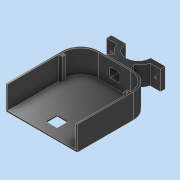
# Autodesk Inventor part: Part2
Saved by Autodesk Inventor 2022 (Build 260153000, 153)
## iProperties
Created: 2022-09-15
Part Number: Part2
Material: Generic
Document SubType Name: Modeling
Designer: aleal
Density: 1 g/cm^3
Appearance: Glossy - Black
Author: aleal
Autodesk Inventor part; units mm, degrees
ref_plane "YZ Plane" through (0, 0, 0) normal (1, 0, 0) x (0, 1, 0)
ref_plane "XZ Plane" through (0, 0, 0) normal (0, 1, 0) x (-1, 0, 0)
sketch "Sketch1" plane through (0, 0, 0) normal (0, 1, 0) x (-1, 0, 0)
  line L0 (0, 0) -> (146, 0)
  line L1 (146, 0) -> (146, -113)
  line L2 (146, -113) -> (0, -113)
  line L3 (0, -113) -> (0, 0)
  dimension "d0" = 146
  dimension "d1" = 113
  constraints: 8 end point, 2 parallel, 1 horizontal, 1 perpendicular
  measures "d0" distance of L1.end L2.end
  measures "d1" distance of L0.end L1.end
extrude "Extrusion1" add sketch "Sketch1" along normal blind 50
sketch "Sketch2" plane through (0, 50, 0) normal (0, 1, 0) x (1, 0, 0)
  line L0 (-146, 0) -> (0, 0) projected
  line L1 (-143, 0) -> (-3, 0)
  line L2 (-3, 0) -> (-3, 72.5)
  line L3 (-40.5, 110) -> (-105.5, 110)
  line L4 (-143, 72.5) -> (-143, 0)
  line L5 (-146, 113) -> (-146, 0) projected
  arc A0 (-105.5, 110) -> (-143, 72.5) centre (-105.5, 72.5) ccw
  arc A1 (-3, 72.5) -> (-40.5, 110) centre (-40.5, 72.5) ccw
  point P0 (-3, 110)
  point P1 (-143, 110)
  dimension "d4" = 140
  dimension "d5" = 110
  dimension "d6" = 3
  dimension "d19" = 37.5
  constraints: 8 end point, 5 point on line, 4 point on circle, 4 tangent, 2 centre point, 2 parallel, 1 equal radius, 1 horizontal, 1 perpendicular
  measures "d4" distance of point (-143, 110) point (-3, 110)
  measures "d5" distance of point (-3, 110) L1.end
  measures "d6" distance between parallel lines of L5 L4
  measures "d19" radius of A0
extrude "Extrusion2" cut sketch "Sketch2" against normal blind 47
ref_plane "Work Plane1" through (0, 45, 0) normal (0, 1, 0) x (1, 0, 0)
sketch "Sketch3" plane through (0, 45, 0) normal (0, 1, 0) x (1, 0, 0)
  arc A0 (-98.4, 158.6) -> (-47.6, 158.6) centre (-73, 158.6) ccw
  line L0 (0, 113) -> (-146, 113) projected
  arc A1 (-108.4, 158.6) -> (-37.6, 158.6) centre (-73, 158.6) ccw
  line L1 (-108.4, 158.6) -> (-98.4, 158.6)
  line L2 (-47.6, 158.6) -> (-37.6, 158.6)
  line L3 (-108.4, 158.6) -> (-128.4, 158.6)
  line L4 (-128.4, 158.6) -> (-128.4, 148.6)
  line L5 (-128.4, 148.6) -> (-106.9582, 148.6)
  line L6 (-37.6, 158.6) -> (-17.6, 158.6)
  line L7 (-17.6, 158.6) -> (-17.6, 148.6)
  line L8 (-17.6, 148.6) -> (-39.0418, 148.6)
  point P0 (0, 0)
  dimension "d10" = 50.8
  dimension "d11" = 45.6
  dimension "d12" = 10
  dimension "d13" = 20
  dimension "d14" = 10
  dimension "d15" = 20
  dimension "d16" = 10
  constraints: 16 end point, 6 point on circle, 4 horizontal, 4 perpendicular, 2 centre point
  measures "d10" diameter of A0
  measures "d11" distance from line of L0 A0.centre
  measures "d12" radial gap between concentric circles of A0 A1
  measures "d13" distance of L1.start L3.end
  measures "d14" distance of L3.end L4.end
  measures "d15" distance of L2.end L6.end
  measures "d16" distance of L6.end L7.end
extrude "Extrusion3" add sketch "Sketch3" against normal blind 40
fillet "Fillet1" radius 37.5 2 edges at (-146, 25, -113) (0, 25, -113)
sketch "Sketch5" plane through (0, 45, 0) normal (0, 1, 0) x (1, 0, 0)
  arc A0 (-106.9582, 148.6) -> (-39.0418, 148.6) centre (-73, 158.6) ccw projected
  line L0 (-37.5, 113) -> (-108.5, 113) projected
  line L1 (-93, 129.3911) -> (-93, 113)
  line L2 (-53, 129.3911) -> (-53, 113)
  point P0 (0, 0)
  constraints: 4 end point, 2 point on circle
extrude "Extrusion4" add sketch "Sketch5" against normal blind 40
fillet "Fillet2" radius 20 2 edges at (-93, 25, -113) (-53, 25, -113)
sketch "Sketch6" plane through (-146, 0, 0) normal (0, 0, 1) x (1, 0, 0)
  line L0 (0, 50) -> (37.5, 50) projected
  line L1 (0, 0) -> (0, 50) projected
  line L2 (0, 50) -> (0, 0)
  line L3 (0, 0) -> (146, 0) projected
  line L4 (0, 0) -> (146, 0)
  line L5 (146, 0) -> (146, 50) projected
  line L6 (146, 0) -> (146, 50)
  line L7 (143, 50) -> (146, 50) projected
  line L8 (146, 50) -> (143, 50)
  line L9 (143, 3) -> (3, 3) projected
  line L10 (143, 50) -> (143, 3)
  line L11 (143, 3) -> (3, 3)
  line L12 (3, 3) -> (3, 50)
  constraints: 14 end point, 4 perpendicular, 3 collinear, 1 point on line
extrude "Extrusion5" add sketch "Sketch6" along normal blind 40
sketch "Sketch7" plane through (-105.5, 50, -110) normal (0, 0, 1) x (1, 0, 0)
  line L0 (42.5, -33.5) -> (22.5, -33.5)
  line L1 (22.5, -33.5) -> (22.5, -13.5)
  line L2 (22.5, -13.5) -> (42.5, -13.5)
  line L3 (42.5, -13.5) -> (42.5, -33.5)
  line L4 (65, 0) -> (65, -47) projected
  line L5 (0, 0) -> (0, -47) projected
  line L6 (0, 0) -> (65, 0) projected
  line L7 (0, -47) -> (65, -47) projected
  point P0 (105.5, -50)
  dimension "d28" = 20
  dimension "d29" = 20
  dimension "d30" = 65
  dimension "d31" = 22.5
  dimension "d32" = 47
  dimension "d33" = 13.5
  constraints: 8 end point, 2 parallel, 1 horizontal, 1 perpendicular
  measures "d28" distance of L1.end L2.end
  measures "d29" distance of L0.end L1.end
  measures "d30" distance between parallel lines of L4 L5
  measures "d31" distance between parallel lines of L4 L3
  measures "d32" distance between parallel lines of L6 L7
  measures "d33" distance between parallel lines of L7 L0
extrude "Extrusion6" cut sketch "Sketch7" against normal blind 30 contours L0 L1 L2 L3
fillet "Fillet3" radius 2 4 edges at (-83, 36.5, -122.6257) (-83, 16.5, -122.6257) (-63, 36.5, -122.6257) (-63, 16.5, -122.6257)
sketch "Sketch8" plane through (0, 50, 0) normal (0, 1, 0) x (1, 0, 0)
  arc A0 (-105.5, 110) -> (-143, 72.5) centre (-105.5, 72.5) ccw projected
  line L0 (-143, 72.5) -> (-136, 72.5)
  line L1 (-136, 72.5) -> (-136, 65.5)
  line L2 (-136, 65.5) -> (-143, 65.5)
  line L3 (-143, 65.5) -> (-143, 72.5)
  arc A1 (-3, 72.5) -> (-40.5, 110) centre (-40.5, 72.5) ccw projected
  line L4 (-3, 72.5) -> (-10, 72.5)
  line L5 (-10, 72.5) -> (-10, 65.5)
  line L6 (-10, 65.5) -> (-3, 65.5)
  line L7 (-3, 65.5) -> (-3, 72.5)
  point P0 (0, 0)
  dimension "d37" = 7
  dimension "d38" = 7
  dimension "d39" = 7
  dimension "d40" = 7
  constraints: 16 end point, 4 parallel, 2 horizontal, 2 perpendicular
  measures "d37" distance of L1.end L2.end
  measures "d38" distance of L0.end L1.end
  measures "d39" distance of L6.end L5.end
  measures "d40" distance of L5.end L4.end
extrude "Extrusion7" add sketch "Sketch8" against normal blind 50
sketch "Sketch9" plane through (0, 50, 0) normal (0, 1, 0) x (1, 0, 0)
  circle A0 centre (-139.5, 69) radius 1.45
  line L0 (-136, 65.5) -> (-136, 72.5) projected
  line L1 (-136, 72.5) -> (-143, 72.5) projected
  circle A1 centre (-6.5, 69) radius 1.45
  line L2 (-10, 72.5) -> (-10, 65.5) projected
  line L3 (-3, 72.5) -> (-10, 72.5) projected
  point P0 (0, 0)
  dimension "d43" = 2.9
  dimension "d44" = 3.5
  dimension "d45" = 3.5
  dimension "d46" = 2.9
  dimension "d47" = 3.5
  dimension "d48" = 3.5
  constraints: 2 centre point
  measures "d43" diameter of A0
  measures "d44" distance from line of L0 A0.centre
  measures "d45" distance from line of L1 A0.centre
  measures "d46" diameter of A1
  measures "d47" distance from line of L2 A1.centre
  measures "d48" distance from line of L3 A1.centre
extrude "Extrusion8" cut sketch "Sketch9" against normal blind 50
sketch "Sketch10" plane through (-98.4, 45, -158.6) normal (0, 0, -1) x (-1, 0, 0)
  circle A0 centre (20, -20) radius 2.75
  circle A1 centre (-70.8, -20) radius 2.75
  line L0 (-50.8, -40) -> (-80.8, -40) projected
  line L1 (30, -40) -> (0, -40) projected
  line L2 (30, 0) -> (30, -40) projected
  line L3 (-80.8, 0) -> (-80.8, -40) projected
  point P0 (-98.4, -45)
  dimension "d54" = 5.5
  dimension "d55" = 5.5
  dimension "d56" = 20
  dimension "d57" = 20
  dimension "d58" = 10
  dimension "d59" = 10
  constraints: 2 centre point
  measures "d54" diameter of A0
  measures "d55" diameter of A1
  measures "d56" distance from line of L0 A1.centre
  measures "d57" distance from line of L1 A0.centre
  measures "d58" distance from line of L2 A0.centre
  measures "d59" distance from line of L3 A1.centre
extrude "Extrusion9" cut sketch "Sketch10" against normal blind 10
sketch "Sketch11" plane through (0, 3, 0) normal (0, 1, 0) x (1, 0, 0)
  line L0 (-84.7, -20) -> (-61.3, -20)
  line L1 (-61.3, -20) -> (-61.3, 3.4)
  line L2 (-61.3, 3.4) -> (-84.7, 3.4)
  line L3 (-84.7, 3.4) -> (-84.7, -20)
  line L4 (-3, 65.5) -> (-3, -40) projected
  line L5 (-143, 65.5) -> (-143, -40) projected
  line L6 (-3, -40) -> (-143, -40) projected
  point P0 (0, 0)
  dimension "d62" = 23.4
  dimension "d63" = 23.4
  dimension "d64" = 140
  dimension "d65" = 58.3
  dimension "d66" = 20
  constraints: 8 end point, 2 parallel, 1 horizontal, 1 perpendicular
  measures "d62" distance of L2.end L1.end
  measures "d63" distance of L1.end L0.end
  measures "d64" distance between parallel lines of L4 L5
  measures "d65" distance between parallel lines of L5 L3
  measures "d66" distance between parallel lines of L6 L0
extrude "Extrusion10" cut sketch "Sketch11" against normal blind 3
equation "\"d31\" = -0.5 * d28 + 0.5 * d30"
equation "\"d33\" = -0.5 * d29 + 0.5 * d32"
equation "\"d65\" = -0.5 * d62 + 0.5 * d64"
body "Solid1"
